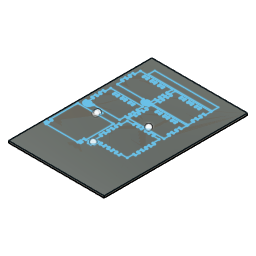
lockable_boxv1 (Autodesk Fusion 360 design; units mm, degrees)
Autodesk Fusion 360 part; units mm, degrees
(part 1 of 2)
box "BoxPrimitive2" add length 225 width 150 height 3 placed x (0, 1, 0) y (-1, 0, 0) z (0, 0, 1) at (150, 0, 0)
sketch "Sketch3" plane through (0, 0, 3) normal (0, 0, 1) x (-1, 0, 0)
  line L0 (-150, -225) -> (0, -225)
  line L1 (0, -225) -> (0, 0)
  line L2 (0, 0) -> (-150, 0)
  line L3 (-150, 0) -> (-150, -225)
  line L4 (-31.0003, -195.1002) -> (-31.0003, -195.1099)
  line L5 (-42.9867, -195.1416) -> (-42.963, -195.1374)
  line L6 (-43.0004, -195.1002) -> (-43.0004, -195.1099)
  line L7 (-36.8003, -195.1002) -> (-36.8003, -192.3001)
  line L8 (-36.8003, -192.3001) -> (-36.8003, -192.289)
  line L9 (-36.8003, -192.3001) -> (-31.0003, -192.3001)
  line L10 (-42.963, -192.2615) -> (-42.9867, -192.2573)
  line L11 (-43.0004, -192.289) -> (-43.0004, -192.3001)
  line L12 (-36.8377, -192.2615) -> (-36.8434, -192.2849)
  line L13 (-42.9591, -195.114) -> (-42.9905, -195.1002)
  line L14 (-45.8995, -195.1002) -> (-48.8004, -195.1002)
  line L15 (-31.0003, -192.289) -> (-31.0003, -192.3001)
  line L16 (-31.0003, -195.1099) -> (-30.9866, -195.1416)
  line L17 (-36.8116, -192.3001) -> (-36.8003, -192.3001)
  line L18 (-31.0003, -192.3001) -> (-30.9908, -192.3001)
  line L19 (-48.8156, -192.2573) -> (-48.8378, -192.2615)
  line L20 (-30.9908, -192.3001) -> (-30.959, -192.2849)
  line L21 (-30.9866, -195.1416) -> (-30.9633, -195.1374)
  line L22 (-36.8003, -195.1099) -> (-36.8003, -195.1002)
  line L23 (-48.8431, -192.2849) -> (-48.8114, -192.3001)
  line L24 (-30.9633, -195.1374) -> (-30.959, -195.114)
  line L25 (-43.0004, -195.1002) -> (-45.8995, -195.1002)
  line L26 (-36.8434, -195.114) -> (-36.8377, -195.1374)
  line L27 (-43.0004, -192.3001) -> (-42.9905, -192.3001)
  line L28 (-59.7005, -61.795) -> (-59.7005, -102.1)
  line L29 (-58.9954, -161.7765) -> (-59.1206, -161.3839)
  line L30 (-60.3306, -156.6707) -> (-60.821, -157.2288)
  line L31 (-61.2359, -157.8504) -> (-61.3297, -158.0117)
  line L32 (-54.2258, -158.6717) -> (-54.0219, -158.9074)
  line L33 (-54.6213, -158.3369) -> (-54.3761, -158.5299)
  line L34 (-59.0433, -159.7508) -> (-58.8807, -159.372)
  line L35 (-54.3761, -158.5299) -> (-54.3002, -158.6015)
  line L36 (-54.3002, -158.6015) -> (-54.2258, -158.6717)
  line L37 (-61.9993, -162.2161) -> (-61.9703, -162.2697)
  line L38 (-53.7905, -159.2492) -> (-53.6113, -159.6214)
  line L39 (-53.6113, -159.6214) -> (-53.5079, -159.9163)
  line L40 (-54.0219, -158.9074) -> (-53.7905, -159.2492)
  line L41 (-57.7536, -158.188) -> (-57.4766, -158.0448)
  line L42 (-58.7996, -162.2104) -> (-58.7996, -162.1995)
  line L43 (-61.9001, -162.3) -> (-58.9001, -162.3)
  line L44 (-12.974, -108.495) -> (-13.679, -108.735)
  line L45 (-6.564, -111.151) -> (-6.657, -110.989)
  line L46 (-16.433, -111.151) -> (-16.527, -111.311)
  line L47 (-16.527, -111.311) -> (-16.764, -111.82)
  line L48 (-6.98, -110.53) -> (-7.47, -109.97)
  line L49 (-5.8, -113.812) -> (-5.85, -113.254)
  line L50 (-8.613, -114.276) -> (-8.68, -114.683)
  line L51 (-8.989, -115.453) -> (-9, -115.488)
  line L52 (-9, -115.501) -> (-9, -115.513)
  line L53 (-8.989, -115.546) -> (-8.986, -115.55)
  line L54 (-8.985, -115.553) -> (-8.955, -115.583)
  line L55 (-8.95, -115.586) -> (-8.947, -115.587)
  line L56 (-8.986, -115.55) -> (-8.985, -115.553)
  line L57 (-9.32, -108.735) -> (-10.024, -108.495)
  line L58 (-8.68, -114.683) -> (-8.806, -115.076)
  line L59 (-8.602, -113.862) -> (-8.598, -113.964)
  line L60 (-8.028, -109.48) -> (-8.489, -109.158)
  line L61 (-8.899, -115.6) -> (-5.899, -115.6)
  line L62 (-8.489, -109.158) -> (-8.649, -109.065)
  line L63 (-63.5839, -109.9) -> (-63.5303, -109.87)
  line L64 (-63.5303, -97.87) -> (-63.5, -97.816)
  line L65 (-63.5, -97.816) -> (-63.5, -97.8)
  line L66 (-63.5303, -109.87) -> (-63.5, -109.816)
  line L67 (-66.5, -91.71) -> (-66.5, -91.7)
  line L68 (-63.5, -85.8) -> (-63.5, -79.8)
  line L69 (-66.5, -85.889) -> (-66.5152, -85.858)
  line L70 (-63.5, -79.8) -> (-63.5, -79.782)
  line L71 (-66.5, -85.9) -> (-66.5, -85.889)
  line L72 (-66.5, -119.8) -> (-66.5, -109.9)
  line L73 (-66.5152, -109.857) -> (-66.537, -109.862)
  line L74 (-63.5839, -97.9) -> (-63.5303, -97.87)
  line L75 (-66.5, -97.9) -> (-63.6005, -97.9)
  line L76 (-66.5109, -103.7) -> (-66.5427, -103.714)
  line L77 (-66.5, -109.889) -> (-66.5152, -109.857)
  line L78 (-66.5, -85.9) -> (-63.6005, -85.9)
  line L79 (-66.5427, -103.714) -> (-66.537, -103.738)
  line L80 (-66.5, -97.889) -> (-66.5152, -97.858)
  line L81 (-66.5152, -97.858) -> (-66.537, -97.862)
  line L82 (-66.5152, -91.742) -> (-66.5, -91.71)
  line L83 (-63.5303, -103.729) -> (-63.5839, -103.7)
  line L84 (-63.6005, -109.9) -> (-63.5839, -109.9)
  line L85 (-66.5427, -97.885) -> (-66.5109, -97.9)
  line L86 (-63.5, -103.782) -> (-63.5303, -103.729)
  line L87 (-66.537, -103.738) -> (-66.5152, -103.742)
  line L88 (-63.6005, -103.7) -> (-66.5, -103.7)
  line L89 (-63.5, -91.8) -> (-63.5, -91.782)
  line L90 (-63.6005, -91.7) -> (-66.5, -91.7)
  line L91 (-82.6629, -119.862) -> (-82.6865, -119.858)
  line L92 (-94.6905, -119.901) -> (-94.6587, -119.886)
  line L93 (-82.6713, -122.8704) -> (-82.6174, -122.9007)
  line L94 (-82.6865, -119.858) -> (-82.7003, -119.89)
  line L95 (-88.5377, -119.862) -> (-88.543, -119.886)
  line L96 (-100.5431, -119.886) -> (-100.5114, -119.901)
  line L97 (-100.583, -122.9007) -> (-100.5293, -122.8704)
  line L98 (-88.5292, -122.8704) -> (-88.5003, -122.8168)
  line L99 (-100.5003, -119.901) -> (-100.5003, -119.89)
  line L100 (-100.5003, -122.8168) -> (-100.5003, -122.8002)
  line L101 (-88.5003, -119.901) -> (-82.7003, -119.901)
  line L102 (-82.5997, -122.9007) -> (-76.5997, -122.9007)
  line L103 (-94.5995, -122.9007) -> (-88.5998, -122.9007)
  line L104 (-106.5995, -122.9007) -> (-100.5996, -122.9007)
  line L105 (-76.5831, -122.9007) -> (-76.5295, -122.8704)
  line L106 (-76.5005, -119.89) -> (-76.5157, -119.858)
  line L107 (-76.5005, -119.901) -> (-76.5005, -119.89)
  line L108 (-76.5157, -119.858) -> (-76.5376, -119.862)
  line L109 (-100.5996, -122.9007) -> (-100.583, -122.9007)
  line L110 (-82.6174, -122.9007) -> (-82.5997, -122.9007)
  line L111 (-63.5303, -91.729) -> (-63.5839, -91.7)
  line L112 (-66.5, -91.7) -> (-66.5109, -91.7)
  line L113 (-63.5, -85.816) -> (-63.5, -85.8)
  line L114 (-63.5, -109.8) -> (-63.5, -103.8)
  line L115 (-63.5, -103.8) -> (-63.5, -103.782)
  line L116 (-66.5427, -109.885) -> (-66.5109, -109.9)
  line L117 (-66.5303, -119.87) -> (-66.5, -119.817)
  line L118 (-66.5, -103.71) -> (-66.5, -103.7)
  line L119 (-82.7003, -122.8168) -> (-82.6713, -122.8704)
  line L120 (-8.806, -115.076) -> (-8.935, -115.36)
  line L121 (-16.341, -110.99) -> (-16.433, -111.151)
  line L122 (-11.686, -108.302) -> (-12.244, -108.35)
  line L123 (-9.197, -112.233) -> (-9.137, -112.317)
  line L124 (-5.899, -115.6) -> (-5.883, -115.6)
  line L125 (-8.829, -162.1293) -> (-8.883, -162.1003)
  line L126 (-8.837, -177.2617) -> (-8.843, -177.285)
  line L127 (-52.8327, -156.1804) -> (-53.2927, -155.8579)
  line L128 (-49.9579, -161.8813) -> (-50.1935, -161.6897)
  line L129 (-50.3851, -161.4526) -> (-50.4155, -161.4004)
  line L130 (-49.5667, -162.052) -> (-49.8521, -161.9434)
  line L131 (-8.837, -171.1375) -> (-8.815, -171.1417)
  line L132 (-49.295, -162.1003) -> (-49.5667, -162.052)
  line L133 (-50.6539, -159.9548) -> (-50.7986, -159.2245)
  line L134 (-50.5576, -161.0614) -> (-50.6042, -160.7898)
  line L135 (-5.829, -171.1293) -> (-5.883, -171.1004)
  line L136 (-5.8, -177.2162) -> (-5.8, -177.1996)
  line L137 (-56.1163, -155.0021) -> (-56.3026, -155.0021)
  line L138 (-53.2927, -155.8579) -> (-53.4529, -155.7655)
  line L139 (-56.3026, -155.0021) -> (-56.4899, -155.0021)
  line L140 (-49.8521, -161.9434) -> (-49.9043, -161.913)
  line L141 (-54.1238, -155.4346) -> (-54.828, -155.1951)
  line L142 (-56.4899, -155.0021) -> (-57.048, -155.0504)
  line L143 (-51.0385, -158.5204) -> (-51.2755, -158.0117)
  line L144 (-50.7986, -159.2245) -> (-51.0385, -158.5204)
  line L145 (-5.829, -177.2698) -> (-5.8, -177.2162)
  line L146 (-5.899, -177.3001) -> (-5.883, -177.3001)
  line L147 (-51.2755, -158.0117) -> (-51.3676, -157.8504)
  line L148 (-57.7769, -155.1951) -> (-58.4824, -155.4346)
  line L149 (-8.899, -162.1003) -> (-49.2044, -162.1003)
  line L150 (-50.6042, -160.7898) -> (-50.6042, -160.7002)
  line L151 (-58.9911, -155.6717) -> (-59.1509, -155.7655)
  line L152 (-50.4472, -161.3465) -> (-50.5576, -161.0614)
  line L153 (-49.2044, -162.1003) -> (-49.295, -162.1003)
  line L154 (-52.2746, -156.6707) -> (-52.8327, -156.1804)
  line L155 (-50.1935, -161.6897) -> (-50.3851, -161.4526)
  line L156 (-58.4824, -155.4346) -> (-58.9911, -155.6717)
  line L157 (-5.883, -171.1004) -> (-5.899, -171.1004)
  line L158 (-53.4529, -155.7655) -> (-53.6155, -155.6717)
  line L159 (-54.828, -155.1951) -> (-55.5582, -155.0504)
  line L160 (-59.1509, -155.7655) -> (-59.3122, -155.8579)
  line L161 (-57.048, -155.0504) -> (-57.7769, -155.1951)
  line L162 (-51.3676, -157.8504) -> (-51.4614, -157.6892)
  line L163 (-8.883, -162.1003) -> (-8.899, -162.1003)
  line L164 (-76.7002, -154.5996) -> (-76.6907, -154.5996)
  line L165 (-82.5115, -157.3999) -> (-82.5433, -157.4137)
  line L166 (-82.5433, -154.5844) -> (-82.5115, -154.5996)
  line L167 (-76.7002, -154.5887) -> (-76.7002, -154.5996)
  line L168 (-76.7002, -157.3999) -> (-76.7002, -157.4095)
  line L169 (-82.5433, -157.4137) -> (-82.5376, -157.437)
  line L170 (-82.5154, -157.4412) -> (-82.5002, -157.4095)
  line L171 (-88.7003, -157.3999) -> (-91.5994, -157.3999)
  line L172 (-76.6865, -157.4412) -> (-76.6632, -157.437)
  line L173 (-63.5, -183.2159) -> (-63.5, -183.1996)
  line L174 (-63.5, -171.1995) -> (-63.5, -162.1995)
  line L175 (-66.5, -177.11) -> (-66.5, -177.1005)
  line L176 (-63.5, -183.1996) -> (-63.5, -177.1996)
  line L177 (-66.537, -171.2616) -> (-66.5427, -171.2849)
  line L178 (-63.5, -162.1995) -> (-63.5, -162.1815)
  line L179 (-63.5839, -162.1003) -> (-63.6005, -162.1003)
  line L180 (-66.5, -183.3002) -> (-63.6005, -183.3002)
  line L181 (-66.5, -189.1003) -> (-66.5, -183.3002)
  line L182 (-66.5152, -177.1417) -> (-66.5, -177.11)
  line L183 (-63.6005, -183.3002) -> (-63.5839, -183.3002)
  line L184 (-66.537, -177.1375) -> (-66.5152, -177.1417)
  line L185 (-119.7005, -162.1995) -> (-119.7005, -171.1995)
  line L186 (-66.5109, -171.3001) -> (-66.5, -171.3001)
  line L187 (-119.7005, -171.2161) -> (-119.6716, -171.2697)
  line L188 (-106.5113, -154.5996) -> (-106.5003, -154.5996)
  line L189 (-116.5999, -162.1003) -> (-119.5999, -162.1003)
  line L190 (-116.7006, -171.3001) -> (-116.6909, -171.3001)
  line L191 (-119.5999, -171.3001) -> (-116.7006, -171.3001)
  line L192 (-100.6905, -154.5996) -> (-100.6588, -154.5844)
  line L193 (-66.5991, -162.1003) -> (-116.5999, -162.1003)
  line L194 (-66.5, -177.1005) -> (-66.5, -171.3001)
  line L195 (-63.5839, -183.3002) -> (-63.5303, -183.2698)
  line L196 (-66.5152, -171.2574) -> (-66.537, -171.2616)
  line L197 (-116.6633, -183.2614) -> (-116.6868, -183.2575)
  line L198 (-116.6909, -189.1003) -> (-116.7006, -189.1003)
  line L199 (-66.5427, -177.1142) -> (-66.537, -177.1375)
  line L200 (-66.5, -183.3002) -> (-66.5, -183.2889)
  line L201 (-66.537, -183.2614) -> (-66.5427, -183.285)
  line L202 (-66.5427, -171.2849) -> (-66.5109, -171.3001)
  line L203 (-63.5303, -183.2698) -> (-63.5, -183.2159)
  line L204 (-66.5109, -183.3002) -> (-66.5, -183.3002)
  line L205 (-106.5003, -154.5996) -> (-100.7001, -154.5996)
  line L206 (-119.6716, -177.1294) -> (-119.7005, -177.1816)
  line L207 (-116.6592, -183.285) -> (-116.6633, -183.2614)
  line L208 (-106.5155, -157.4412) -> (-106.5003, -157.4095)
  line L209 (-119.7005, -189.1815) -> (-119.7005, -189.1995)
  line L210 (-119.7005, -183.1996) -> (-119.7005, -183.2159)
  line L211 (-100.7001, -154.5887) -> (-100.7001, -154.5996)
  line L212 (-106.5155, -154.5569) -> (-106.5375, -154.5625)
  line L213 (-63.5839, -177.1005) -> (-63.6005, -177.1005)
  line L214 (-119.7005, -171.1995) -> (-119.7005, -171.2161)
  line L215 (-116.7006, -183.2889) -> (-116.7006, -183.3002)
  line L216 (-66.5, -183.2889) -> (-66.5152, -183.2575)
  line L217 (-63.5, -171.2161) -> (-63.5, -171.1995)
  line L218 (-100.7001, -154.5996) -> (-100.7001, -157.3999)
  line L219 (-100.6588, -154.5844) -> (-100.6629, -154.5625)
  line L220 (-63.5, -162.1815) -> (-63.5303, -162.1293)
  line L221 (-119.6716, -162.1293) -> (-119.7005, -162.1815)
  line L222 (-100.7001, -157.3999) -> (-100.7001, -157.4095)
  line L223 (-116.7006, -177.1005) -> (-119.5999, -177.1005)
  line L224 (-106.543, -154.5844) -> (-106.5113, -154.5996)
  line L225 (-116.6909, -183.3002) -> (-116.6592, -183.285)
  line L226 (-63.6005, -171.3001) -> (-63.5839, -171.3001)
  line L227 (-119.7005, -162.1815) -> (-119.7005, -162.1995)
  line L228 (-63.6005, -177.1005) -> (-66.5, -177.1005)
  line L229 (-63.6005, -162.1003) -> (-66.5991, -162.1003)
  line L230 (-63.5, -177.1996) -> (-63.5, -177.1816)
  line L231 (-116.6592, -189.114) -> (-116.6909, -189.1003)
  line L232 (-100.6864, -154.5569) -> (-100.7001, -154.5887)
  line L233 (-66.5, -171.3001) -> (-66.5, -171.2891)
  line L234 (-66.5, -177.1005) -> (-66.5109, -177.1005)
  line L235 (-119.6179, -171.3001) -> (-119.5999, -171.3001)
  line L236 (-119.6179, -162.1003) -> (-119.6716, -162.1293)
  line L237 (-66.5427, -183.285) -> (-66.5109, -183.3002)
  line L238 (-100.6864, -157.4412) -> (-100.6629, -157.437)
  line L239 (-100.6629, -154.5625) -> (-100.6864, -154.5569)
  line L240 (-116.6909, -177.1005) -> (-116.7006, -177.1005)
  line L241 (-100.7001, -154.5996) -> (-100.6905, -154.5996)
  line L242 (-119.7005, -189.1995) -> (-119.7005, -198.1994)
  line L243 (-106.5003, -157.4095) -> (-106.5003, -157.3999)
  line L244 (-119.7005, -177.1816) -> (-119.7005, -177.1996)
  line L245 (-119.6716, -189.1292) -> (-119.7005, -189.1815)
  line L246 (-100.6629, -157.437) -> (-100.6588, -157.4137)
  line L247 (-119.6179, -177.1005) -> (-119.6716, -177.1294)
  line L248 (-106.5003, -157.3999) -> (-106.5113, -157.3999)
  line L249 (-119.6179, -198.3) -> (-119.5999, -198.3)
  line L250 (-116.7006, -189.1099) -> (-116.6868, -189.1416)
  line L251 (-106.5375, -157.437) -> (-106.5155, -157.4412)
  line L252 (-106.543, -157.4137) -> (-106.5375, -157.437)
  line L253 (-106.5003, -154.5996) -> (-106.5003, -154.5887)
  line L254 (-116.7006, -189.1003) -> (-119.5999, -189.1003)
  line L255 (-100.7001, -157.4095) -> (-100.6864, -157.4412)
  line L256 (-119.7005, -183.2159) -> (-119.6716, -183.2698)
  line L257 (-116.6868, -189.1416) -> (-116.6633, -189.1374)
  line L258 (-106.5375, -154.5625) -> (-106.543, -154.5844)
  line L259 (-119.6179, -183.3002) -> (-119.5999, -183.3002)
  line L260 (-116.6633, -189.1374) -> (-116.6592, -189.114)
  line L261 (-119.7005, -198.216) -> (-119.6716, -198.2697)
  line L262 (-103.5996, -157.3999) -> (-106.5003, -157.3999)
  line L263 (-119.5999, -183.3002) -> (-116.7006, -183.3002)
  line L264 (-119.5999, -198.3) -> (-116.5999, -198.3)
  line L265 (-116.6592, -177.1142) -> (-116.6909, -177.1005)
  line L266 (-119.6716, -198.2697) -> (-119.6179, -198.3)
  line L267 (-106.5003, -157.3999) -> (-106.5003, -154.5996)
  line L268 (-116.7006, -189.1003) -> (-116.7006, -189.1099)
  line L269 (-116.6633, -177.1375) -> (-116.6592, -177.1142)
  line L270 (-106.5003, -154.5887) -> (-106.5155, -154.5569)
  line L271 (-119.5999, -177.1005) -> (-119.6179, -177.1005)
  line L272 (-119.7005, -198.1994) -> (-119.7005, -198.216)
  line L273 (-119.6179, -189.1003) -> (-119.6716, -189.1292)
  line L274 (-106.5113, -157.3999) -> (-106.543, -157.4137)
  line L275 (-119.6716, -183.2698) -> (-119.6179, -183.3002)
  line L276 (-116.6868, -183.2575) -> (-116.7006, -183.2889)
  line L277 (-116.7006, -183.3002) -> (-116.6909, -183.3002)
  line L278 (-119.5999, -189.1003) -> (-119.6179, -189.1003)
  line L279 (-116.7006, -183.3002) -> (-116.7006, -189.1003)
  line L280 (-119.7005, -177.1996) -> (-119.7005, -183.1996)
  line L281 (-94.543, -157.4137) -> (-94.5377, -157.437)
  line L282 (-82.5002, -157.3999) -> (-82.5002, -154.5996)
  line L283 (-82.5002, -154.5996) -> (-82.5002, -154.5887)
  line L284 (-94.543, -154.5844) -> (-94.5113, -154.5996)
  line L285 (-94.5003, -154.5887) -> (-94.5155, -154.5569)
  line L286 (-82.5002, -157.4095) -> (-82.5002, -157.3999)
  line L287 (-88.6904, -154.5996) -> (-88.6587, -154.5844)
  line L288 (-82.5002, -157.3999) -> (-82.5115, -157.3999)
  line L289 (-82.5376, -157.437) -> (-82.5154, -157.4412)
  line L290 (-76.6589, -154.5844) -> (-76.6632, -154.5625)
  line L291 (-76.6865, -154.5569) -> (-76.7002, -154.5887)
  line L292 (-88.6629, -157.437) -> (-88.6587, -157.4137)
  line L293 (-88.7003, -154.5996) -> (-88.7003, -157.3999)
  line L294 (-82.5154, -154.5569) -> (-82.5376, -154.5625)
  line L295 (-94.5003, -157.4095) -> (-94.5003, -157.3999)
  line L296 (-100.6588, -157.4137) -> (-100.6905, -157.3999)
  line L297 (-94.5155, -154.5569) -> (-94.5377, -154.5625)
  line L298 (-88.7003, -154.5996) -> (-88.6904, -154.5996)
  line L299 (-88.6629, -154.5625) -> (-88.6865, -154.5569)
  line L300 (-94.5377, -154.5625) -> (-94.543, -154.5844)
  line L301 (-94.5113, -154.5996) -> (-94.5003, -154.5996)
  line L302 (-94.5003, -154.5996) -> (-88.7003, -154.5996)
  line L303 (-82.5002, -154.5996) -> (-76.7002, -154.5996)
  line L304 (-79.5997, -157.3999) -> (-82.5002, -157.3999)
  line L305 (-63.5839, -124.4) -> (-63.6005, -124.4)
  line L306 (-119.7005, -124.4826) -> (-119.7005, -124.5006)
  line L307 (-66.5, -139.3998) -> (-66.5109, -139.3998)
  line L308 (-66.5, -133.5998) -> (-63.6005, -133.5998)
  line L309 (-63.5, -124.4826) -> (-63.5303, -124.429)
  line L310 (-66.5991, -124.4) -> (-116.5999, -124.4)
  line L311 (-66.5427, -151.4137) -> (-66.537, -151.4369)
  line L312 (-66.5, -139.3998) -> (-66.5, -133.5998)
  line L313 (-66.537, -139.4372) -> (-66.5152, -139.4414)
  line L314 (-63.5303, -133.5709) -> (-63.5, -133.5172)
  line L315 (-63.6005, -145.5999) -> (-63.5839, -145.5999)
  line L316 (-63.5, -160.5171) -> (-63.5, -160.5005)
  line L317 (-66.5109, -145.5999) -> (-66.5, -145.5999)
  line L318 (-66.5, -145.5999) -> (-63.6005, -145.5999)
  line L319 (-66.5152, -151.4412) -> (-66.5, -151.4094)
  line L320 (-63.5303, -160.5707) -> (-63.5, -160.5171)
  line L321 (-63.5, -133.5172) -> (-63.5, -133.5006)
  line L322 (-63.6005, -133.5998) -> (-63.5839, -133.5998)
  line L323 (-66.5152, -145.5568) -> (-66.537, -145.5625)
  line L324 (-63.5839, -145.5999) -> (-63.5303, -145.5709)
  line L325 (-63.5, -139.4827) -> (-63.5303, -139.4287)
  line L326 (-63.5303, -139.4287) -> (-63.5839, -139.3998)
  line L327 (-66.5427, -139.4136) -> (-66.537, -139.4372)
  line L328 (-119.7005, -124.5006) -> (-119.7005, -133.5006)
  line L329 (-66.5, -151.3999) -> (-66.5, -145.5999)
  line L330 (-66.537, -151.4369) -> (-66.5152, -151.4412)
  line L331 (-66.5, -151.4094) -> (-66.5, -151.3999)
  line L332 (-63.5839, -151.3999) -> (-63.6005, -151.3999)
  line L333 (-63.5839, -139.3998) -> (-63.6005, -139.3998)
  line L334 (-63.5, -151.4824) -> (-63.5303, -151.4288)
  line L335 (-63.5, -145.517) -> (-63.5, -145.5004)
  line L336 (-66.5427, -133.5846) -> (-66.5109, -133.5998)
  line L337 (-63.5839, -133.5998) -> (-63.5303, -133.5709)
  line L338 (-63.5, -151.5004) -> (-63.5, -151.4824)
  line L339 (-63.6005, -139.3998) -> (-66.5, -139.3998)
  line L340 (-63.5, -160.5005) -> (-63.5, -151.5004)
  line L341 (-63.5, -139.5003) -> (-63.5, -139.4827)
  line L342 (-66.5152, -133.5571) -> (-66.537, -133.5624)
  line L343 (-66.537, -133.5624) -> (-66.5427, -133.5846)
  line L344 (-66.5109, -133.5998) -> (-66.5, -133.5998)
  line L345 (-66.5152, -139.4414) -> (-66.5, -139.4097)
  line L346 (-63.5839, -160.5996) -> (-63.5303, -160.5707)
  line L347 (-63.5, -133.5006) -> (-63.5, -124.5006)
  line L348 (-66.5109, -151.3999) -> (-66.5427, -151.4137)
  line L349 (-66.5427, -145.5847) -> (-66.5109, -145.5999)
  line L350 (-63.6005, -151.3999) -> (-66.5, -151.3999)
  line L351 (-63.6005, -124.4) -> (-66.5991, -124.4)
  line L352 (-63.5, -145.5004) -> (-63.5, -139.5003)
  line L353 (-66.5, -133.5888) -> (-66.5152, -133.5571)
  line L354 (-106.6712, -122.8704) -> (-106.6174, -122.9007)
  line L355 (-119.6716, -139.4287) -> (-119.7005, -139.4827)
  line L356 (-119.6716, -145.5709) -> (-119.6179, -145.5999)
  line L357 (-106.6864, -119.858) -> (-106.7001, -119.89)
  line L358 (-106.7001, -119.89) -> (-106.7001, -119.901)
  line L359 (-116.7006, -145.5999) -> (-116.6909, -145.5999)
  line L360 (-116.6592, -139.4136) -> (-116.6909, -139.3998)
  line L361 (-119.5999, -145.5999) -> (-116.7006, -145.5999)
  line L362 (-116.6633, -151.4369) -> (-116.6592, -151.4137)
  line L363 (-119.5999, -133.5998) -> (-116.7006, -133.5998)
  line L364 (-116.6633, -145.5625) -> (-116.6868, -145.5568)
  line L365 (-119.7005, -151.4824) -> (-119.7005, -151.5004)
  line L366 (-119.7005, -139.5003) -> (-119.7005, -145.5004)
  line L367 (-116.6868, -133.5571) -> (-116.7006, -133.5888)
  line L368 (-119.6179, -160.5996) -> (-119.5999, -160.5996)
  line L369 (-106.7001, -122.8002) -> (-106.7001, -122.8168)
  line L370 (-106.7001, -122.8168) -> (-106.6712, -122.8704)
  line L371 (-116.6909, -145.5999) -> (-116.6592, -145.5847)
  line L372 (-116.7006, -133.5998) -> (-116.6909, -133.5998)
  line L373 (-119.6716, -133.5709) -> (-119.6179, -133.5998)
  line L374 (-116.7006, -139.4097) -> (-116.6868, -139.4414)
  line L375 (-119.6179, -145.5999) -> (-119.5999, -145.5999)
  line L376 (-116.7006, -139.3998) -> (-116.7006, -139.4097)
  line L377 (-106.7001, -119.901) -> (-106.7001, -122.8002)
  line L378 (-116.6592, -151.4137) -> (-116.6909, -151.3999)
  line L379 (-116.6868, -151.4412) -> (-116.6633, -151.4369)
  line L380 (-119.7005, -133.5172) -> (-119.6716, -133.5709)
  line L381 (-116.6633, -133.5624) -> (-116.6868, -133.5571)
  line L382 (-119.7005, -145.517) -> (-119.6716, -145.5709)
  line L383 (-116.7006, -139.3998) -> (-119.5999, -139.3998)
  line L384 (-119.7005, -145.5004) -> (-119.7005, -145.517)
  line L385 (-116.7006, -145.5886) -> (-116.7006, -145.5999)
  line L386 (-116.7006, -151.4094) -> (-116.6868, -151.4412)
  line L387 (-116.7006, -145.5999) -> (-116.7006, -151.3999)
  line L388 (-116.6868, -139.4414) -> (-116.6633, -139.4372)
  line L389 (-116.6909, -139.3998) -> (-116.7006, -139.3998)
  line L390 (-116.6592, -145.5847) -> (-116.6633, -145.5625)
  line L391 (-116.6909, -151.3999) -> (-116.7006, -151.3999)
  line L392 (-116.7006, -133.5888) -> (-116.7006, -133.5998)
  line L393 (-119.7005, -151.5004) -> (-119.7005, -160.5005)
  line L394 (-116.6909, -133.5998) -> (-116.6592, -133.5846)
  line L395 (-119.6179, -151.3999) -> (-119.6716, -151.4288)
  line L396 (-119.5999, -151.3999) -> (-119.6179, -151.3999)
  line L397 (-88.7003, -157.4095) -> (-88.6865, -157.4412)
  line L398 (-94.5003, -157.3999) -> (-94.5113, -157.3999)
  line L399 (-94.5377, -157.437) -> (-94.5155, -157.4412)
  line L400 (-88.6865, -154.5569) -> (-88.7003, -154.5887)
  line L401 (-76.6632, -154.5625) -> (-76.6865, -154.5569)
  line L402 (-76.7002, -154.5996) -> (-76.7002, -157.3999)
  line L403 (-76.6589, -157.4137) -> (-76.6907, -157.3999)
  line L404 (-76.6907, -157.3999) -> (-76.7002, -157.3999)
  line L405 (-82.5002, -154.5887) -> (-82.5154, -154.5569)
  line L406 (-88.6587, -157.4137) -> (-88.6904, -157.3999)
  line L407 (-88.7003, -154.5887) -> (-88.7003, -154.5996)
  line L408 (-100.7001, -157.3999) -> (-103.5996, -157.3999)
  line L409 (-116.5999, -160.5996) -> (-66.5991, -160.5996)
  line L410 (-88.7003, -157.3999) -> (-88.7003, -157.4095)
  line L411 (-88.6904, -157.3999) -> (-88.7003, -157.3999)
  line L412 (-94.5155, -157.4412) -> (-94.5003, -157.4095)
  line L413 (-82.5376, -154.5625) -> (-82.5433, -154.5844)
  line L414 (-100.6905, -157.3999) -> (-100.7001, -157.3999)
  line L415 (-76.7002, -157.3999) -> (-79.5997, -157.3999)
  line L416 (-91.5994, -157.3999) -> (-94.5003, -157.3999)
  line L417 (-63.6005, -160.5996) -> (-63.5839, -160.5996)
  line L418 (-94.5003, -157.3999) -> (-94.5003, -154.5996)
  line L419 (-82.5115, -154.5996) -> (-82.5002, -154.5996)
  line L420 (-66.5991, -160.5996) -> (-63.6005, -160.5996)
  line L421 (-88.6865, -157.4412) -> (-88.6629, -157.437)
  line L422 (-88.6587, -154.5844) -> (-88.6629, -154.5625)
  line L423 (-76.6907, -154.5996) -> (-76.6589, -154.5844)
  line L424 (-94.5003, -154.5996) -> (-94.5003, -154.5887)
  line L425 (-94.5113, -157.3999) -> (-94.543, -157.4137)
  line L426 (-76.7002, -157.4095) -> (-76.6865, -157.4412)
  line L427 (-76.6632, -157.437) -> (-76.6589, -157.4137)
  line L428 (-66.5, -133.5998) -> (-66.5, -133.5888)
  line L429 (-63.5303, -124.429) -> (-63.5839, -124.4)
  line L430 (-66.5, -145.5886) -> (-66.5152, -145.5568)
  line L431 (-116.5999, -124.4) -> (-119.5999, -124.4)
  line L432 (-66.5109, -139.3998) -> (-66.5427, -139.4136)
  line L433 (-66.537, -145.5625) -> (-66.5427, -145.5847)
  line L434 (-119.5999, -124.4) -> (-119.6179, -124.4)
  line L435 (-119.6716, -124.429) -> (-119.7005, -124.4826)
  line L436 (-63.5, -124.5006) -> (-63.5, -124.4826)
  line L437 (-66.5, -151.3999) -> (-66.5109, -151.3999)
  line L438 (-66.5, -139.4097) -> (-66.5, -139.3998)
  line L439 (-63.5303, -145.5709) -> (-63.5, -145.517)
  line L440 (-63.5303, -151.4288) -> (-63.5839, -151.3999)
  line L441 (-119.6179, -124.4) -> (-119.6716, -124.429)
  line L442 (-66.5, -145.5999) -> (-66.5, -145.5886)
  line L443 (-5.829, -183.1291) -> (-5.883, -183.1002)
  line L444 (-24.838, -192.2615) -> (-24.843, -192.2849)
  line L445 (-8.8, -177.2892) -> (-8.815, -177.2574)
  line L446 (-24.812, -195.1002) -> (-24.843, -195.114)
  line L447 (-19, -192.3001) -> (-19, -195.1002)
  line L448 (-5.8, -183.1816) -> (-5.829, -183.1291)
  line L449 (-18.959, -192.2849) -> (-18.963, -192.2615)
  line L450 (-24.816, -192.2573) -> (-24.838, -192.2615)
  line L451 (-24.801, -195.1002) -> (-24.812, -195.1002)
  line L452 (-24.801, -192.3001) -> (-19, -192.3001)
  line L453 (-8.815, -183.1418) -> (-8.8, -183.11)
  line L454 (-5.883, -183.1002) -> (-5.899, -183.1002)
  line L455 (-8.8, -183.1002) -> (-8.811, -183.1002)
  line L456 (-8.811, -183.1002) -> (-8.843, -183.1139)
  line L457 (-24.801, -192.289) -> (-24.816, -192.2573)
  line L458 (-18.986, -195.1416) -> (-18.963, -195.1374)
  line L459 (-24.801, -195.1099) -> (-24.801, -195.1002)
  line L460 (-24.843, -192.2849) -> (-24.812, -192.3001)
  line L461 (-8.815, -189.2574) -> (-8.837, -189.2615)
  line L462 (-24.801, -195.1002) -> (-24.801, -192.3001)
  line L463 (-61.9001, -142.5999) -> (-58.9992, -142.5999)
  line L464 (-61.9993, -142.5004) -> (-61.9993, -142.5169)
  line L465 (-61.9181, -142.5999) -> (-61.9001, -142.5999)
  line L466 (-8.8, -198.216) -> (-8.8, -198.1994)
  line L467 (-8.8, -189.3001) -> (-5.899, -189.3001)
  line L468 (-8.883, -198.3) -> (-8.829, -198.2697)
  line L469 (-5.883, -189.3001) -> (-5.829, -189.2697)
  line L470 (-5.8, -183.1996) -> (-5.8, -183.1816)
  line L471 (-24.812, -192.3001) -> (-24.801, -192.3001)
  line L472 (-18.986, -192.2573) -> (-19, -192.289)
  line L473 (-21.9, -195.1002) -> (-24.801, -195.1002)
  line L474 (-19, -192.3001) -> (-18.991, -192.3001)
  line L475 (-18.963, -195.1374) -> (-18.959, -195.114)
  line L476 (-58.9001, -198.3) -> (-8.899, -198.3)
  line L477 (-18.991, -195.1002) -> (-19, -195.1002)
  line L478 (-5.8, -189.216) -> (-5.8, -189.1995)
  line L479 (-8.8, -189.3001) -> (-8.8, -189.289)
  line L480 (-8.8, -198.1994) -> (-8.8, -189.3001)
  line L481 (-8.811, -189.3001) -> (-8.8, -189.3001)
  line L482 (-24.816, -195.1416) -> (-24.801, -195.1099)
  line L483 (-30.959, -195.114) -> (-30.9908, -195.1002)
  line L484 (-19, -195.1099) -> (-18.986, -195.1416)
  line L485 (-82.659, -119.886) -> (-82.6629, -119.862)
  line L486 (-100.5003, -119.89) -> (-100.5155, -119.858)
  line L487 (-88.5116, -119.901) -> (-88.5003, -119.901)
  line L488 (-100.5003, -122.8002) -> (-100.5003, -119.901)
  line L489 (-88.543, -119.886) -> (-88.5116, -119.901)
  line L490 (-82.7003, -119.901) -> (-82.7003, -122.8002)
  line L491 (-119.7005, -160.5005) -> (-119.7005, -160.5171)
  line L492 (-116.7006, -151.3999) -> (-119.5999, -151.3999)
  line L493 (-119.7005, -160.5171) -> (-119.6716, -160.5707)
  line L494 (-116.6633, -139.4372) -> (-116.6592, -139.4136)
  line L495 (-119.6716, -160.5707) -> (-119.6179, -160.5996)
  line L496 (-116.6592, -133.5846) -> (-116.6633, -133.5624)
  line L497 (-119.6179, -133.5998) -> (-119.5999, -133.5998)
  line L498 (-116.7006, -151.3999) -> (-116.7006, -151.4094)
  line L499 (-119.5999, -160.5996) -> (-116.5999, -160.5996)
  line L500 (-119.6716, -151.4288) -> (-119.7005, -151.4824)
  line L501 (-116.7006, -133.5998) -> (-116.7006, -139.3998)
  line L502 (-119.7005, -133.5006) -> (-119.7005, -133.5172)
  line L503 (-106.7001, -119.901) -> (-106.6905, -119.901)
  line L504 (-106.6588, -119.886) -> (-106.6629, -119.862)
  line L505 (-106.6905, -119.901) -> (-106.6588, -119.886)
  line L506 (-116.5999, -119.901) -> (-106.7001, -119.901)
  line L507 (-116.6868, -145.5568) -> (-116.7006, -145.5886)
  line L508 (-106.6629, -119.862) -> (-106.6864, -119.858)
  line L509 (-119.6179, -139.3998) -> (-119.6716, -139.4287)
  line L510 (-119.7005, -139.4827) -> (-119.7005, -139.5003)
  line L511 (-76.5376, -119.862) -> (-76.5432, -119.886)
  line L512 (-94.6862, -119.858) -> (-94.7, -119.89)
  line L513 (-76.5115, -119.901) -> (-76.5005, -119.901)
  line L514 (-88.5003, -119.901) -> (-88.5003, -119.89)
  line L515 (-100.5376, -119.862) -> (-100.5431, -119.886)
  line L516 (-82.7003, -122.8002) -> (-82.7003, -122.8168)
  line L517 (-94.7, -122.8168) -> (-94.6711, -122.8704)
  line L518 (-119.5999, -139.3998) -> (-119.6179, -139.3998)
  line L519 (-76.5295, -122.8704) -> (-76.5005, -122.8168)
  line L520 (-94.6174, -122.9007) -> (-94.5995, -122.9007)
  line L521 (-82.7003, -119.901) -> (-82.6907, -119.901)
  line L522 (-94.7, -122.8002) -> (-94.7, -122.8168)
  line L523 (-76.5997, -122.9007) -> (-76.5831, -122.9007)
  line L524 (-100.5155, -119.858) -> (-100.5376, -119.862)
  line L525 (-76.5005, -122.8168) -> (-76.5005, -122.8002)
  line L526 (-94.7, -119.901) -> (-94.7, -122.8002)
  line L527 (-76.5432, -119.886) -> (-76.5115, -119.901)
  line L528 (-76.5005, -119.901) -> (-66.5991, -119.901)
  line L529 (-94.7, -119.89) -> (-94.7, -119.901)
  line L530 (-82.7003, -119.89) -> (-82.7003, -119.901)
  line L531 (-100.5114, -119.901) -> (-100.5003, -119.901)
  line L532 (-100.5003, -119.901) -> (-94.7, -119.901)
  line L533 (-76.5005, -122.8002) -> (-76.5005, -119.901)
  line L534 (-66.5991, -119.901) -> (-66.5825, -119.901)
  line L535 (-66.5825, -119.901) -> (-66.5303, -119.87)
  line L536 (-94.663, -119.862) -> (-94.6862, -119.858)
  line L537 (-100.5293, -122.8704) -> (-100.5003, -122.8168)
  line L538 (-94.6587, -119.886) -> (-94.663, -119.862)
  line L539 (-106.6174, -122.9007) -> (-106.5995, -122.9007)
  line L540 (-94.7, -119.901) -> (-94.6905, -119.901)
  line L541 (-88.5998, -122.9007) -> (-88.5832, -122.9007)
  line L542 (-88.5003, -122.8168) -> (-88.5003, -122.8002)
  line L543 (-88.5832, -122.9007) -> (-88.5292, -122.8704)
  line L544 (-88.5003, -122.8002) -> (-88.5003, -119.901)
  line L545 (-94.6711, -122.8704) -> (-94.6174, -122.9007)
  line L546 (-88.5154, -119.858) -> (-88.5377, -119.862)
  line L547 (-82.6907, -119.901) -> (-82.659, -119.886)
  line L548 (-88.5003, -119.89) -> (-88.5154, -119.858)
  line L549 (-56.7006, -52.1) -> (-56.7006, -53.298)
  line L550 (-56.7006, -53.308) -> (-56.6868, -53.34)
  line L551 (-56.6909, -56.097) -> (-56.6592, -56.082)
  line L552 (-48.8114, -192.3001) -> (-48.8004, -192.3001)
  line L553 (-48.8004, -195.1099) -> (-48.8004, -195.1002)
  line L554 (-43.0004, -195.1099) -> (-42.9867, -195.1416)
  line L555 (-59.7005, -105.117) -> (-59.6716, -105.17)
  line L556 (-59.7005, -105.1) -> (-59.7005, -105.117)
  line L557 (-59.7005, -102.1) -> (-59.7005, -105.1)
  line L558 (-48.8004, -192.289) -> (-48.8156, -192.2573)
  line L559 (-48.8004, -195.1002) -> (-48.8004, -192.3001)
  line L560 (-42.9591, -192.2849) -> (-42.963, -192.2615)
  line L561 (-42.9905, -192.3001) -> (-42.9591, -192.2849)
  line L562 (-59.5999, -105.199) -> (-56.5999, -105.199)
  line L563 (-59.6716, -105.17) -> (-59.6179, -105.199)
  line L564 (-42.9867, -192.2573) -> (-43.0004, -192.289)
  line L565 (-48.8156, -195.1416) -> (-48.8004, -195.1099)
  line L566 (-3.5839, -53.298) -> (-3.6005, -53.298)
  line L567 (-59.6179, -56.097) -> (-59.5999, -56.097)
  line L568 (-56.6633, -53.336) -> (-56.6592, -53.312)
  line L569 (-56.6179, -52) -> (-56.6716, -52.029)
  line L570 (-56.7006, -61.696) -> (-59.5999, -61.696)
  line L571 (-6.5, -52.082) -> (-6.5303, -52.029)
  line L572 (-3.5, -56.013) -> (-3.5, -55.997)
  line L573 (-56.6633, -61.733) -> (-56.6592, -61.71)
  line L574 (-56.6633, -56.058) -> (-56.6868, -56.055)
  line L575 (-59.5999, -56.097) -> (-56.7006, -56.097)
  line L576 (-59.7005, -56.013) -> (-59.6716, -56.067)
  line L577 (-59.5999, -61.696) -> (-59.6179, -61.696)
  line L578 (-59.6179, -61.696) -> (-59.6716, -61.725)
  line L579 (-56.6909, -53.298) -> (-56.7006, -53.298)
  line L580 (-6.5427, -56.082) -> (-6.5109, -56.097)
  line L581 (-56.6592, -53.312) -> (-56.6909, -53.298)
  line L582 (-3.5, -53.399) -> (-3.5, -53.381)
  line L583 (-6.537, -53.336) -> (-6.5152, -53.34)
  line L584 (-59.7005, -55.997) -> (-59.7005, -56.013)
  line L585 (-59.6179, -53.298) -> (-59.6716, -53.327)
  line L586 (-6.5109, -56.097) -> (-6.5, -56.097)
  line L587 (-6.5427, -53.312) -> (-6.537, -53.336)
  line L588 (-6.5, -53.298) -> (-6.5109, -53.298)
  line L589 (-56.6909, -61.696) -> (-56.7006, -61.696)
  line L590 (-3.6005, -53.298) -> (-6.5, -53.298)
  line L591 (-56.6592, -56.082) -> (-56.6633, -56.058)
  line L592 (-3.5, -55.997) -> (-3.5, -53.399)
  line L593 (-3.5839, -56.097) -> (-3.5303, -56.067)
  line L594 (-56.7006, -56.097) -> (-56.7006, -61.696)
  line L595 (-6.5, -53.298) -> (-6.5, -52.1)
  line L596 (-6.5825, -52) -> (-6.5991, -52)
  line L597 (-6.5303, -52.029) -> (-6.5825, -52)
  line L598 (-6.5, -53.308) -> (-6.5, -53.298)
  line L599 (-3.6005, -56.097) -> (-3.5839, -56.097)
  line L600 (-56.6868, -53.34) -> (-56.6633, -53.336)
  line L601 (-59.6716, -53.327) -> (-59.7005, -53.381)
  line L602 (-59.6716, -56.067) -> (-59.6179, -56.097)
  line L603 (-3.5303, -53.327) -> (-3.5839, -53.298)
  line L604 (-56.5999, -52) -> (-56.6179, -52)
  line L605 (-56.7006, -53.298) -> (-59.5999, -53.298)
  line L606 (-56.7006, -56.097) -> (-56.6909, -56.097)
  line L607 (-6.5, -56.097) -> (-3.6005, -56.097)
  line L608 (-6.5991, -52) -> (-56.5999, -52)
  line L609 (-56.6716, -52.029) -> (-56.7006, -52.082)
  line L610 (-6.5, -52.1) -> (-6.5, -52.082)
  line L611 (-59.5999, -53.298) -> (-59.6179, -53.298)
  line L612 (-59.7005, -53.381) -> (-59.7005, -53.399)
  line L613 (-3.5, -53.381) -> (-3.5303, -53.327)
  line L614 (-3.5303, -56.067) -> (-3.5, -56.013)
  line L615 (-6.5152, -53.34) -> (-6.5, -53.308)
  line L616 (-59.7005, -53.399) -> (-59.7005, -55.997)
  line L617 (-56.7006, -53.298) -> (-56.7006, -53.308)
  line L618 (-8.982, -115.441) -> (-8.986, -115.45)
  line L619 (-12.576, -116.693) -> (-12.948, -116.512)
  line L620 (-61.9181, -183.1002) -> (-61.9703, -183.1291)
  line L621 (-55.1021, -159.1885) -> (-55.1021, -159.1995)
  line L622 (-57.5123, -161.9998) -> (-57.544, -162.0136)
  line L623 (-58.958, -183.1139) -> (-58.9897, -183.1002)
  line L624 (-57.5013, -162.0093) -> (-57.5013, -161.9998)
  line L625 (-61.9993, -189.216) -> (-61.9703, -189.2697)
  line L626 (-61.9001, -183.1002) -> (-61.9181, -183.1002)
  line L627 (-58.958, -189.2849) -> (-58.9622, -189.2615)
  line L628 (-58.9855, -183.1418) -> (-58.9622, -183.1375)
  line L629 (-61.9993, -183.1816) -> (-61.9993, -183.1996)
  line L630 (-57.5165, -162.0411) -> (-57.5013, -162.0093)
  line L631 (-61.9993, -183.1996) -> (-61.9993, -189.1995)
  line L632 (-61.9703, -183.1291) -> (-61.9993, -183.1816)
  line L633 (-55.0926, -159.1995) -> (-55.0608, -159.1843)
  line L634 (-61.9703, -189.2697) -> (-61.9181, -189.3001)
  line L635 (-57.544, -162.0136) -> (-57.5387, -162.0368)
  line L636 (-57.5013, -161.9998) -> (-57.5123, -161.9998)
  line L637 (-55.1021, -159.1995) -> (-55.1021, -161.9998)
  line L638 (-58.9992, -198.1994) -> (-58.9992, -198.216)
  line L639 (-58.9181, -198.3) -> (-58.9001, -198.3)
  line L640 (-58.9897, -189.3001) -> (-58.958, -189.2849)
  line L641 (-55.0926, -161.9998) -> (-55.1021, -161.9998)
  line L642 (-58.9992, -189.289) -> (-58.9992, -189.3001)
  line L643 (-56.3026, -159.1995) -> (-55.1021, -159.1995)
  line L644 (-55.1021, -162.0093) -> (-55.0883, -162.0411)
  line L645 (-55.0651, -162.0368) -> (-55.0608, -162.0136)
  line L646 (-58.9703, -198.2697) -> (-58.9181, -198.3)
  line L647 (-55.0608, -159.1843) -> (-55.0651, -159.1624)
  line L648 (-58.9992, -189.3001) -> (-58.9897, -189.3001)
  line L649 (-58.9622, -189.2615) -> (-58.9855, -189.2574)
  line L650 (-58.9992, -189.3001) -> (-58.9992, -198.1994)
  line L651 (-61.9001, -189.3001) -> (-58.9992, -189.3001)
  line L652 (-55.1021, -159.1995) -> (-55.0926, -159.1995)
  line L653 (-55.0608, -162.0136) -> (-55.0926, -161.9998)
  line L654 (-57.5387, -162.0368) -> (-57.5165, -162.0411)
  line L655 (-57.5013, -159.1995) -> (-57.5013, -159.1885)
  line L656 (-57.5013, -161.9998) -> (-57.5013, -159.1995)
  line L657 (-55.1021, -161.9998) -> (-57.5013, -161.9998)
  line L658 (-58.9622, -183.1375) -> (-58.958, -183.1139)
  line L659 (-57.5165, -159.1568) -> (-57.5387, -159.1624)
  line L660 (-57.5013, -159.1885) -> (-57.5165, -159.1568)
  line L661 (-61.9181, -189.3001) -> (-61.9001, -189.3001)
  line L662 (-58.9855, -189.2574) -> (-58.9992, -189.289)
  line L663 (-58.9992, -183.1002) -> (-61.9001, -183.1002)
  line L664 (-58.9992, -198.216) -> (-58.9703, -198.2697)
  line L665 (-55.0883, -162.0411) -> (-55.0651, -162.0368)
  line L666 (-8.8, -130.5998) -> (-5.899, -130.5998)
  line L667 (-5.8, -130.5172) -> (-5.8, -130.5006)
  line L668 (-55.0883, -159.1568) -> (-55.1021, -159.1885)
  line L669 (-19, -148.3999) -> (-21.9, -148.3999)
  line L670 (-19, -148.3999) -> (-19, -148.4094)
  line L671 (-8.8, -151.5004) -> (-8.8, -142.5999)
  line L672 (-8.843, -124.4138) -> (-8.837, -124.4371)
  line L673 (-18.963, -148.4373) -> (-18.959, -148.4136)
  line L674 (-18.991, -148.3999) -> (-19, -148.3999)
  line L675 (-8.8, -142.5886) -> (-8.815, -142.5572)
  line L676 (-8.8, -142.5999) -> (-5.899, -142.5999)
  line L677 (-5.8, -142.5004) -> (-5.8, -136.5007)
  line L678 (-5.8, -136.4827) -> (-5.829, -136.4287)
  line L679 (-8.811, -124.4) -> (-8.843, -124.4138)
  line L680 (-58.9001, -151.5996) -> (-8.899, -151.5996)
  line L681 (-5.8, -124.5006) -> (-5.8, -124.4826)
  line L682 (-18.986, -145.5568) -> (-19, -145.5886)
  line L683 (-58.9897, -183.1002) -> (-58.9992, -183.1002)
  line L684 (-5.883, -130.5998) -> (-5.829, -130.5708)
  line L685 (-8.8, -124.4) -> (-8.811, -124.4)
  line L686 (-61.9993, -189.1995) -> (-61.9993, -189.216)
  line L687 (-55.0651, -159.1624) -> (-55.0883, -159.1568)
  line L688 (-58.9992, -183.11) -> (-58.9855, -183.1418)
  line L689 (-8.811, -136.3998) -> (-8.843, -136.4135)
  line L690 (-8.8, -151.517) -> (-8.8, -151.5004)
  line L691 (-8.837, -130.5627) -> (-8.843, -130.5846)
  line L692 (-19, -145.5886) -> (-19, -145.5999)
  line L693 (-5.829, -124.429) -> (-5.883, -124.4)
  line L694 (-18.959, -148.4136) -> (-18.991, -148.3999)
  line L695 (-8.8, -136.3998) -> (-8.8, -130.5998)
  line L696 (-5.899, -142.5999) -> (-5.883, -142.5999)
  line L697 (-5.883, -142.5999) -> (-5.829, -142.5709)
  line L698 (-8.837, -142.5625) -> (-8.843, -142.5847)
  line L699 (-8.843, -142.5847) -> (-8.811, -142.5999)
  line L700 (-8.899, -151.5996) -> (-8.883, -151.5996)
  line L701 (-8.829, -151.5706) -> (-8.8, -151.517)
  line L702 (-5.899, -130.5998) -> (-5.883, -130.5998)
  line L703 (-5.8, -136.5007) -> (-5.8, -136.4827)
  line L704 (-8.843, -136.4135) -> (-8.837, -136.4372)
  line L705 (-5.8, -130.5006) -> (-5.8, -124.5006)
  line L706 (-18.963, -145.5625) -> (-18.986, -145.5568)
  line L707 (-5.883, -136.3998) -> (-5.899, -136.3998)
  line L708 (-5.883, -124.4) -> (-5.899, -124.4)
  line L709 (-5.829, -142.5709) -> (-5.8, -142.5169)
  line L710 (-8.815, -142.5572) -> (-8.837, -142.5625)
  line L711 (-5.8, -142.5169) -> (-5.8, -142.5004)
  line L712 (-5.8, -124.4826) -> (-5.829, -124.429)
  line L713 (-5.829, -130.5708) -> (-5.8, -130.5172)
  line L714 (-8.8, -136.3998) -> (-8.811, -136.3998)
  line L715 (-5.899, -124.4) -> (-8.8, -124.4)
  line L716 (-8.837, -136.4372) -> (-8.815, -136.4414)
  line L717 (-8.883, -151.5996) -> (-8.829, -151.5706)
  line L718 (-12.448, -111.259) -> (-12.149, -111.172)
  line L719 (-13.179, -111.637) -> (-12.827, -111.422)
  line L720 (-8.8, -136.4097) -> (-8.8, -136.3998)
  line L721 (-5.829, -136.4287) -> (-5.883, -136.3998)
  line L722 (-8.843, -130.5846) -> (-8.811, -130.5998)
  line L723 (-8.8, -130.5888) -> (-8.815, -130.5571)
  line L724 (-19, -148.4094) -> (-18.986, -148.4411)
  line L725 (-12.047, -111.153) -> (-11.946, -111.132)
  line L726 (-8.8, -130.5998) -> (-8.8, -130.5888)
  line L727 (-8.815, -130.5571) -> (-8.837, -130.5627)
  line L728 (-14.075, -115.328) -> (-14.205, -115.044)
  line L729 (-14.395, -114.138) -> (-14.385, -113.724)
  line L730 (-18.986, -148.4411) -> (-18.963, -148.4373)
  line L731 (-5.899, -136.3998) -> (-8.8, -136.3998)
  line L732 (-8.811, -142.5999) -> (-8.8, -142.5999)
  line L733 (-19, -145.5999) -> (-19, -148.3999)
  line L734 (-8.815, -136.4414) -> (-8.8, -136.4097)
  line L735 (-8.8, -142.5999) -> (-8.8, -142.5886)
  line L736 (-8.811, -130.5998) -> (-8.8, -130.5998)
  line L737 (-13.425, -111.83) -> (-13.179, -111.637)
  line L738 (-10.517, -111.269) -> (-10.421, -111.307)
  line L739 (-9.497, -116.099) -> (-9.816, -116.362)
  line L740 (-14.385, -113.724) -> (-14.341, -113.416)
  line L741 (-14.205, -115.044) -> (-14.238, -114.948)
  line L742 (-10.049, -111.488) -> (-9.707, -111.719)
  line L743 (-13.779, -112.207) -> (-13.575, -111.971)
  line L744 (-14.316, -113.316) -> (-14.293, -113.216)
  line L745 (-10.95, -116.847) -> (-11.359, -116.895)
  line L746 (-10.816, -111.18) -> (-10.517, -111.269)
  line L747 (-13.372, -116.215) -> (-13.599, -115.999)
  line L748 (-13.291, -116.279) -> (-13.372, -116.215)
  line L749 (-14.272, -114.85) -> (-14.345, -114.547)
  line L750 (-14.011, -112.549) -> (-13.779, -112.207)
  line L751 (-10.55, -116.739) -> (-10.95, -116.847)
  line L752 (-14.191, -112.921) -> (-14.011, -112.549)
  line L753 (-9.038, -115.538) -> (-9.219, -115.793)
  line L754 (-8.8, -124.4) -> (-8.8, -115.501)
  line L755 (-13.599, -115.999) -> (-13.862, -115.681)
  line L756 (-9.707, -111.719) -> (-9.401, -111.998)
  line L757 (-9.401, -111.998) -> (-9.197, -112.233)
  line L758 (-9.219, -115.793) -> (-9.497, -116.099)
  line L759 (-12.827, -111.422) -> (-12.448, -111.259)
  line L760 (-10.326, -111.344) -> (-10.049, -111.488)
  line L761 (-11.223, -111.112) -> (-10.816, -111.18)
  line L762 (-8.921, -115.4) -> (-8.982, -115.441)
  line L763 (-8.8, -124.4096) -> (-8.8, -124.4)
  line L764 (-11.877, -116.877) -> (-12.183, -116.818)
  line L765 (-8.815, -124.4413) -> (-8.8, -124.4096)
  line L766 (-14.345, -114.547) -> (-14.395, -114.138)
  line L767 (-11.636, -111.102) -> (-11.223, -111.112)
  line L768 (-12.948, -116.512) -> (-13.211, -116.343)
  line L769 (-13.211, -116.343) -> (-13.291, -116.279)
  line L770 (-11.774, -116.887) -> (-11.877, -116.877)
  line L771 (-11.946, -111.132) -> (-11.636, -111.102)
  line L772 (-12.183, -116.818) -> (-12.576, -116.693)
  line L773 (-10.168, -116.578) -> (-10.261, -116.625)
  line L774 (-11.359, -116.895) -> (-11.672, -116.896)
  line L775 (-10.421, -111.307) -> (-10.326, -111.344)
  line L776 (-8.8, -115.501) -> (-8.8, -115.483)
  line L777 (-9.816, -116.362) -> (-10.077, -116.53)
  line L778 (-13.499, -111.901) -> (-13.425, -111.83)
  line L779 (-8.8, -115.483) -> (-8.829, -115.429)
  line L780 (-14.293, -113.216) -> (-14.191, -112.921)
  line L781 (-12.149, -111.172) -> (-12.047, -111.153)
  line L782 (-8.986, -115.45) -> (-9.038, -115.538)
  line L783 (-88.7003, -192.3001) -> (-88.7003, -195.1002)
  line L784 (-82.5002, -195.1002) -> (-82.5002, -192.3001)
  line L785 (-116.6909, -171.3001) -> (-116.6592, -171.2849)
  line L786 (-76.6632, -192.2615) -> (-76.6865, -192.2573)
  line L787 (-116.7006, -171.3001) -> (-116.7006, -177.1005)
  line L788 (-63.5, -189.1995) -> (-63.5, -189.1815)
  line L789 (-82.5115, -192.3001) -> (-82.5002, -192.3001)
  line L790 (-82.5002, -195.1002) -> (-82.5115, -195.1002)
  line L791 (-116.6633, -171.2616) -> (-116.6868, -171.2574)
  line L792 (-63.5, -198.216) -> (-63.5, -198.1994)
  line L793 (-63.5303, -171.2697) -> (-63.5, -171.2161)
  line L794 (-66.5, -171.2891) -> (-66.5152, -171.2574)
  line L795 (-63.5, -177.1816) -> (-63.5303, -177.1294)
  line L796 (-76.6589, -195.114) -> (-76.6907, -195.1002)
  line L797 (-63.5303, -162.1293) -> (-63.5839, -162.1003)
  line L798 (-82.5002, -192.3001) -> (-82.5002, -192.289)
  line L799 (-66.537, -189.1374) -> (-66.5152, -189.1416)
  line L800 (-116.7006, -177.1005) -> (-116.7006, -177.11)
  line L801 (-63.5839, -171.3001) -> (-63.5303, -171.2697)
  line L802 (-82.5433, -195.114) -> (-82.5376, -195.1374)
  line L803 (-63.5839, -198.3) -> (-63.5303, -198.2697)
  line L804 (-82.5376, -195.1374) -> (-82.5154, -195.1416)
  line L805 (-79.5997, -195.1002) -> (-82.5002, -195.1002)
  line L806 (-82.5433, -192.2849) -> (-82.5115, -192.3001)
  line L807 (-76.7002, -195.1099) -> (-76.6865, -195.1416)
  line L808 (-63.5303, -189.1292) -> (-63.5839, -189.1003)
  line L809 (-88.6587, -195.114) -> (-88.6904, -195.1002)
  line L810 (-116.6868, -171.2574) -> (-116.7006, -171.2891)
  line L811 (-66.5, -171.3001) -> (-63.6005, -171.3001)
  line L812 (-119.5999, -162.1003) -> (-119.6179, -162.1003)
  line L813 (-116.6592, -171.2849) -> (-116.6633, -171.2616)
  line L814 (-63.5303, -177.1294) -> (-63.5839, -177.1005)
  line L815 (-76.7002, -195.1002) -> (-79.5997, -195.1002)
  line L816 (-116.6868, -177.1417) -> (-116.6633, -177.1375)
  line L817 (-66.5152, -183.2575) -> (-66.537, -183.2614)
  line L818 (-88.6865, -192.2573) -> (-88.7003, -192.289)
  line L819 (-66.5, -189.1003) -> (-66.5109, -189.1003)
  line L820 (-66.5152, -189.1416) -> (-66.5, -189.1099)
  line L821 (-63.5, -189.1815) -> (-63.5303, -189.1292)
  line L822 (-63.5303, -198.2697) -> (-63.5, -198.216)
  line L823 (-66.5, -189.1099) -> (-66.5, -189.1003)
  line L824 (-82.5154, -192.2573) -> (-82.5376, -192.2615)
  line L825 (-76.7002, -195.1002) -> (-76.7002, -195.1099)
  line L826 (-82.5002, -192.289) -> (-82.5154, -192.2573)
  line L827 (-76.6632, -195.1374) -> (-76.6589, -195.114)
  line L828 (-88.7003, -195.1002) -> (-88.7003, -195.1099)
  line L829 (-76.6907, -195.1002) -> (-76.7002, -195.1002)
  line L830 (-116.7006, -171.2891) -> (-116.7006, -171.3001)
  line L831 (-66.5991, -198.3) -> (-63.6005, -198.3)
  line L832 (-119.6716, -171.2697) -> (-119.6179, -171.3001)
  line L833 (-116.7006, -177.11) -> (-116.6868, -177.1417)
  line L834 (-88.7003, -192.289) -> (-88.7003, -192.3001)
  line L835 (-66.5109, -177.1005) -> (-66.5427, -177.1142)
  line L836 (-88.7003, -195.1099) -> (-88.6865, -195.1416)
  line L837 (-88.6865, -195.1416) -> (-88.6629, -195.1374)
  line L838 (-88.6904, -195.1002) -> (-88.7003, -195.1002)
  line L839 (-66.5109, -189.1003) -> (-66.5427, -189.114)
  line L840 (-88.6629, -195.1374) -> (-88.6587, -195.114)
  line L841 (-76.6865, -195.1416) -> (-76.6632, -195.1374)
  line L842 (-116.5999, -198.3) -> (-66.5991, -198.3)
  line L843 (-76.6589, -192.2849) -> (-76.6632, -192.2615)
  line L844 (-82.5002, -192.3001) -> (-76.7002, -192.3001)
  line L845 (-82.5115, -195.1002) -> (-82.5433, -195.114)
  line L846 (-66.5427, -189.114) -> (-66.537, -189.1374)
  line L847 (-76.7002, -192.3001) -> (-76.6907, -192.3001)
  line L848 (-30.9908, -148.3999) -> (-31.0003, -148.3999)
  line L849 (-31.0003, -148.3999) -> (-33.8998, -148.3999)
  line L850 (-30.959, -148.4136) -> (-30.9908, -148.3999)
  line L851 (-30.9866, -148.4411) -> (-30.9633, -148.4373)
  line L852 (-30.9633, -148.4373) -> (-30.959, -148.4136)
  line L853 (-43.0004, -148.3999) -> (-45.8995, -148.3999)
  line L854 (-48.8378, -148.4373) -> (-48.8156, -148.4411)
  line L855 (-57.5013, -159.1995) -> (-56.3026, -159.1995)
  line L856 (-45.8995, -148.3999) -> (-48.8004, -148.3999)
  line L857 (-24.801, -148.3999) -> (-24.812, -148.3999)
  line L858 (-48.8004, -148.3999) -> (-48.8004, -145.5999)
  line L859 (-42.9905, -145.5999) -> (-42.9591, -145.5847)
  line L860 (-36.8003, -145.5999) -> (-36.8003, -145.5886)
  line L861 (-43.0004, -145.5886) -> (-43.0004, -145.5999)
  line L862 (-36.8155, -145.5568) -> (-36.8377, -145.5625)
  line L863 (-31.0003, -148.3999) -> (-31.0003, -148.4094)
  line L864 (-57.5123, -159.1995) -> (-57.5013, -159.1995)
  line L865 (-48.8378, -145.5625) -> (-48.8431, -145.5847)
  line L866 (-42.963, -145.5625) -> (-42.9867, -145.5568)
  line L867 (-30.9866, -145.5568) -> (-31.0003, -145.5886)
  line L868 (-24.816, -148.4411) -> (-24.801, -148.4094)
  line L869 (-31.0003, -145.5886) -> (-31.0003, -145.5999)
  line L870 (-57.5387, -159.1624) -> (-57.544, -159.1843)
  line L871 (-30.9908, -145.5999) -> (-30.959, -145.5847)
  line L872 (-31.0003, -145.5999) -> (-31.0003, -148.3999)
  line L873 (-24.843, -145.5847) -> (-24.812, -145.5999)
  line L874 (-43.0004, -148.4094) -> (-42.9867, -148.4411)
  line L875 (-48.8431, -148.4136) -> (-48.8378, -148.4373)
  line L876 (-48.8156, -148.4411) -> (-48.8004, -148.4094)
  line L877 (-48.8156, -145.5568) -> (-48.8378, -145.5625)